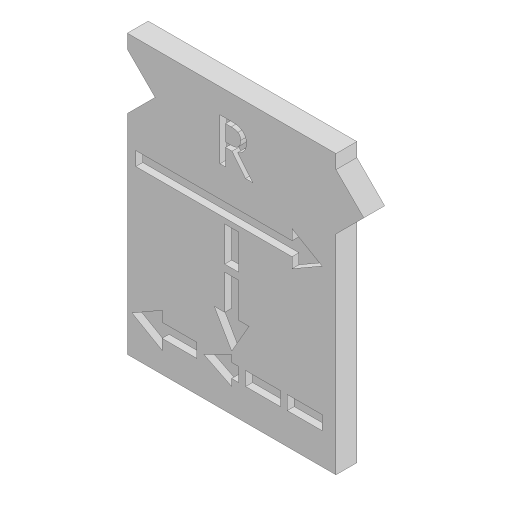
# Autodesk Inventor part: MS_R[202] text
Saved by Autodesk Inventor 2023 (Build 270158000, 158)
## iProperties
Created: 2023-03-29
Part Number: MS_R[202] text
Material: Generic
Document SubType Name: Modeling
Designer: LKLM8608
Density: 1 g/cm^3
Appearance: Default
Author: LKLM8608
Autodesk Inventor part; units mm, degrees
ref_plane "YZ Plane" through (0, 0, 0) normal (1, 0, 0) x (0, 1, 0)
ref_plane "XZ Plane" through (0, 0, 0) normal (0, 1, 0) x (-1, 0, 0)
ref_plane "XY Plane" through (0, 0, 0) normal (0, 0, 1) x (1, 0, 0)
sketch "Sketch1" plane through (0, 0, 0) normal (0, 0, 1) x (1, 0, 0)
  line L0 (0, 0) -> (-30, 0)
  line L1 (-30, 40) -> (0, 40)
  line L2 (-36.1318, 34) -> (13.8682, 34) construction
  circle A0 centre (0, 34) radius 4 construction
  circle A1 centre (-30, 34) radius 4 construction
  line L3 (-30, 30) -> (0, 30) construction
  line L4 (0, 30) -> (4, 34)
  line L5 (4, 34) -> (0, 38)
  line L6 (-30, 30) -> (-26, 34)
  line L7 (-26, 34) -> (-30, 38)
  line L8 (-30, 0) -> (-30, 30)
  line L9 (-30, 38) -> (-30, 40)
  line L10 (0, 40) -> (0, 38)
  line L11 (0, 30) -> (0, 0)
  dimension "d0" = 30
  dimension "d1" = 40
  dimension "d2" = 50
  dimension "d3" = 6
  dimension "d4" = 8
  dimension "d5" = 8
  constraints: 24 end point, 6 point on circle, 5 parallel, 4 perpendicular, 3 point on line, 2 centre point, 2 horizontal
  measures "d0" distance of L1.start L1.end
  measures "d1" distance of L0.end L1.start
  measures "d2" distance of L2.start L2.end
  measures "d3" distance between parallel lines of L2 L1
  measures "d4" diameter of A0
  measures "d5" diameter of A1
extrude "Extrusion1" add sketch "Sketch1" along normal blind 3
sketch "Sketch2" plane through (0, 0, 3) normal (0, 0, 1) x (1, 0, 0)
  line L0 (-30, 30) -> (-30, 0) construction
  line L1 (-30, 0) -> (0, 0) construction
  line L2 (0, 0) -> (0, 30) construction
  line L3 (-17.303, 36.5) -> (-11.9002, 36.5) construction
  line L4 (-11.9002, 36.5) -> (-11.9002, 30.2072) construction
  line L5 (-11.9002, 30.2072) -> (-17.303, 30.2072) construction
  line L6 (-17.303, 30.2072) -> (-17.303, 36.5) construction
  line L7 (-28.7886, 24) -> (-6.3197, 24)
  line L8 (-6.3197, 24) -> (-6.3197, 26)
  line L9 (-6.3197, 26) -> (-28.7886, 26)
  line L10 (-30, 25) -> (0, 25) construction
  line L11 (-6.3197, 26) -> (-6.3197, 27.5)
  line L12 (-6.3197, 27.5) -> (-1.9896, 25)
  line L13 (-6.3197, 24) -> (-6.3197, 22.5)
  line L14 (-6.3197, 22.5) -> (-1.9896, 25)
  line L15 (-16, 12.2406) -> (-17.5, 12.2406)
  line L16 (-17.5, 12.2406) -> (-15, 7.9105)
  line L17 (-14, 12.2406) -> (-12.5, 12.2406)
  line L18 (-12.5, 12.2406) -> (-15, 7.9105)
  line L19 (-30, 5.5) -> (0, 5.5) construction
  line L20 (-6.9986, 6.5) -> (-1.9986, 6.5)
  line L21 (-1.9986, 6.5) -> (-1.9986, 4.5)
  line L22 (-1.9986, 4.5) -> (-6.9986, 4.5)
  line L23 (-6.9986, 4.5) -> (-6.9986, 6.5)
  line L24 (-6.9986, 6.5) -> (-1.9986, 4.5) construction
  line L25 (-1.9986, 6.5) -> (-6.9986, 4.5) construction
  line L26 (-1.9896, 25) -> (-1.9896, 0) construction
  line L27 (-12.9986, 6.5) -> (-7.9986, 6.5)
  line L28 (-36, 5.5) -> (-6, 5.5) construction
  line L29 (-7.9986, 4.5) -> (-12.9986, 4.5)
  line L30 (-12.9986, 4.5) -> (-12.9986, 6.5)
  line L31 (-7.9986, 6.5) -> (-7.9986, 4.5)
  line L32 (-18.9986, 6.5) -> (-13.9986, 6.5)
  line L33 (-42, 5.5) -> (-12, 5.5) construction
  line L34 (-13.9986, 4.5) -> (-18.9986, 4.5)
  line L35 (-18.9986, 4.5) -> (-18.9986, 5.4478)
  line L36 (-13.9986, 6.5) -> (-13.9986, 4.5)
  line L37 (-24.9986, 6.5) -> (-19.9986, 6.5)
  line L38 (-48, 5.5) -> (-18, 5.5) construction
  line L39 (-19.9986, 4.5) -> (-24.9986, 4.5)
  line L40 (-24.9986, 4.5) -> (-24.9986, 6.5)
  line L41 (-19.9986, 6.5) -> (-19.9986, 4.5)
  line L42 (-24.9986, 6.5) -> (-24.9986, 8)
  line L43 (-24.9986, 8) -> (-29.3287, 5.5)
  line L44 (-24.9986, 4.5) -> (-24.9986, 3)
  line L45 (-24.9986, 3) -> (-29.3287, 5.5)
  line L46 (-28.7886, 26) -> (-28.7886, 24)
  line L47 (-15, 6.5) -> (-15, 7.5)
  line L48 (-15, 7.5) -> (-18.9986, 5.5)
  line L49 (-15, 4.5) -> (-15, 3.5)
  line L50 (-15, 3.5) -> (-18.9986, 5.5)
  line L51 (-15, 6.5) -> (-13.9986, 6.5)
  line L52 (-13.9986, 6.5) -> (-13.9986, 4.5)
  line L53 (-13.9986, 4.5) -> (-15, 4.5)
  line L54 (-15, -0.4455) -> (-15, 27.9265) construction
  line L55 (-16, 12.2406) -> (-16, 17.2406)
  line L56 (-14, 17.2406) -> (-14, 12.2406)
  line L57 (-16, 18.2406) -> (-14, 18.2406)
  line L58 (-14, 18.2406) -> (-14, 23.2406)
  line L59 (-14, 23.2406) -> (-16, 23.2406)
  line L60 (-16, 23.2406) -> (-16, 18.2406)
  line L61 (-16, 17.2406) -> (-14, 17.2406)
  line L62 (0, 40) -> (-30, 40) construction
  line L63 (-11.9643, 30.4) -> (-13.0172, 30.4)
  line L64 (-13.0172, 30.4) -> (-14.9451, 32.8271)
  line L65 (-14.9451, 32.8271) -> (-15.8744, 32.8271)
  line L66 (-15.8744, 32.8271) -> (-15.8744, 30.4)
  line L67 (-15.8744, 30.4) -> (-16.6851, 30.4)
  line L68 (-16.6851, 30.4) -> (-16.6851, 36.5)
  line L69 (-16.6851, 36.5) -> (-15.1132, 36.5)
  spline S0 degree 2 poles (-15.1132, 36.5) (-14.5892, 36.5) (-13.8823, 36.3863) (-13.561, 36.1787) knots 0 0 0 1 2 2 2
  spline S1 degree 2 poles (-13.561, 36.1787) (-13.2397, 35.9711) (-12.8689, 35.3235) (-12.8689, 34.844) knots 0 0 0 1 2 2 2
  spline S2 degree 2 poles (-12.8689, 34.844) (-12.8689, 34.1767) (-13.5511, 33.272) (-14.1344, 33.0545) knots 0 0 0 1 2 2 2
  line L70 (-14.1344, 33.0545) -> (-11.9643, 30.4)
  spline S3 degree 2 poles (-13.7142, 34.7797) (-13.7142, 35.0467) (-13.9021, 35.457) (-14.0998, 35.5904) knots 0 0 0 1 2 2 2
  spline S4 degree 2 poles (-14.0998, 35.5904) (-14.2728, 35.7041) (-14.7325, 35.7981) (-15.0687, 35.7981) knots 0 0 0 1 2 2 2
  line L71 (-15.0687, 35.7981) -> (-15.8744, 35.7981)
  line L72 (-15.8744, 35.7981) -> (-15.8744, 33.5044)
  line L73 (-15.8744, 33.5044) -> (-15.1626, 33.5044)
  spline S5 degree 2 poles (-15.1626, 33.5044) (-14.8116, 33.5044) (-14.253, 33.628) (-14.0602, 33.8207) knots 0 0 0 1 2 2 2
  spline S6 degree 2 poles (-14.0602, 33.8207) (-13.8823, 33.9888) (-13.7142, 34.4634) (-13.7142, 34.7797) knots 0 0 0 1 2 2 2
  point P0 (-30, 24.9574)
  point P1 (-4.4986, 5.5)
  point P2 (-10.4986, 5.5)
  point P3 (-16.4986, 5.5)
  point P4 (-22.4986, 5.5)
  point P5 (-15, 7.9105)
  point P6 (-15, 18.2406)
  point P7 (-15, 40)
  dimension "d18" = 1.5
  dimension "d19" = 5
  dimension "d20" = 1.5
  dimension "d21" = 1.5
  dimension "d22" = 5
  dimension "d23" = 1.5
  dimension "d24" = 5
  dimension "d25" = 2
  dimension "d28" = 6
  dimension "d33" = 1.5
  dimension "d34" = 5
  dimension "d35" = 1.5
  dimension "d38" = 1
  dimension "d39" = 1
  dimension "d40" = 25
  dimension "d41" = 1
  dimension "d42" = 1
  dimension "d43" = 5
  dimension "d44" = 2
  dimension "d45" = 5
  dimension "d47" = 1
  dimension "d48" = 8
  dimension "d49" = 3.5
  constraints: 110 end point, 15 point on line, 12 perpendicular, 6 horizontal, 4 midpoint, 4 parallel, 3 collinear, 3 vertical, 37 other
  measures "d18" distance of L8.end L11.end
  measures "d19" distance of L11.end L12.end
  measures "d20" distance of L7.end L13.end
  measures "d21" distance of L15.start L15.end
  measures "d22" distance of L15.end L16.end
  measures "d23" distance of L17.start L17.end
  measures "d24" distance of L21.end L22.end
  measures "d25" distance of L20.end L21.end
  measures "d28" distance of L20.start L27.start
  measures "d33" distance of L37.start L42.end
  measures "d34" distance of L42.end L43.end
  measures "d35" distance of L39.end L44.end
  measures "d38" distance of L47.start L47.end
  measures "d39" distance of L49.start L49.end
  measures "d40" distance from line of L26.end L10
  measures "d41" distance between parallel lines of L9 L10
  measures "d42" distance from line of L7.start L10
  measures "d43" distance of L15.start L55.end
  measures "d44" distance of L55.end L56.start
  measures "d45" distance of L57.end L58.end
  measures "d47" distance between parallel lines of L57 L61
  measures "d48" distance from line of L42.end L1
  measures "d49" distance from line of point (-15, 40) L3
extrude "Extrusion2" cut sketch "Sketch2" against normal blind 1
body "Solid1"
